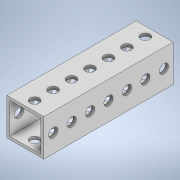
# Autodesk Inventor part: SquareTube
Saved by Autodesk Inventor 2020 (Build 240168000, 168)
## iProperties
Created: 2021-11-12
Part Number: SquareTube
Material: Generic
Document SubType Name: Modeling
Designer: 17185
Density: 1 g/cm^3
Appearance: Default
Author: 17185
Autodesk Inventor part; units mm, degrees
ref_plane "YZ Plane" through (0, 0, 0) normal (1, 0, 0) x (0, 1, 0)
ref_plane "XZ Plane" through (0, 0, 0) normal (0, 1, 0) x (-1, 0, 0)
ref_plane "XY Plane" through (0, 0, 0) normal (0, 0, 1) x (1, 0, 0)
sketch "Sketch1" plane through (0, 0, 0) normal (0, 0, 1) x (1, 0, 0)
  line L0 (-12.7, 12.7) -> (12.7, 12.7)
  line L1 (12.7, 12.7) -> (12.7, -12.7)
  line L2 (12.7, -12.7) -> (-12.7, -12.7)
  line L3 (-12.7, -12.7) -> (-12.7, 12.7)
  line L4 (-12.7, 12.7) -> (12.7, -12.7) construction
  line L5 (12.7, 12.7) -> (-12.7, -12.7) construction
  point P0 (0, 0)
  dimension "d0" = 25.4
  dimension "d1" = 25.4
  constraints: 12 end point, 2 midpoint, 2 parallel, 1 horizontal, 1 perpendicular
  measures "d0" distance of L0.end L1.end
  measures "d1" distance of L1.end L2.end
extrude "Extrusion1" add sketch "Sketch1" along normal blind 88.9
shell "Shell1" thickness 1.9844 removed faces 2 at (4.2333, -4.2333, 0) at (4.2333, -4.2333, 88.9)
sketch "Sketch2" plane through (-12.7, -12.7, 0) normal (-1, 0, 0) x (0, 0, 1)
  circle A0 centre (19.0501, 12.7399) radius 3.175
  circle A1 centre (31.7501, 12.7399) radius 3.175
  line L0 (0, 12.7) -> (88.9, 12.7) construction
  circle A2 centre (44.45, 12.7) radius 3.175
  circle A3 centre (57.15, 12.7) radius 3.175
  circle A4 centre (69.85, 12.7) radius 3.175
  circle A5 centre (82.55, 12.7) radius 3.175
  line L1 (0, 25.4) -> (88.9, 25.4) construction
  line L2 (44.45, 25.4) -> (44.45, 0) construction
  circle A6 centre (6.3501, 12.7) radius 3.175
  dimension "d5" = 6.35
  dimension "d6" = 6.35
  dimension "d7" = 6.35
  dimension "d8" = 6.35
  dimension "d9" = 6.35
  dimension "d10" = 6.35
  dimension "d11" = 12.7
  dimension "d12" = 12.7
  dimension "d13" = 12.7
  dimension "d14" = 12.7
  dimension "d15" = 12.7
  dimension "d16" = 6.35
  dimension "d17" = 12.7
  constraints: 7 centre point, 4 end point, 4 point on line, 3 midpoint, 1 horizontal, 1 vertical
  measures "d5" diameter of A0
  measures "d6" diameter of A1
  measures "d7" diameter of A2
  measures "d8" diameter of A3
  measures "d9" diameter of A4
  measures "d10" diameter of A5
  measures "d11" distance of A1.centre A0.centre
  measures "d12" distance of A2.centre A1.centre
  measures "d13" distance of A2.centre A3.centre
  measures "d14" distance of A4.centre A3.centre
  measures "d15" distance of A5.centre A4.centre
  measures "d16" diameter of A6
  measures "d17" distance of A6.centre A0.centre
extrude "Extrusion2" cut sketch "Sketch2" against normal blind 88.9
sketch "Sketch3" plane through (-12.7, 12.7, 0) normal (0, 1, 0) x (1, 0, 0)
  line L0 (23.4156, -47.625) -> (25.4, -47.625) construction
  circle A0 centre (12.7, -44.45) radius 3.175
  circle A1 centre (12.7, -31.75) radius 3.175
  circle A2 centre (12.7, -19.05) radius 3.175
  circle A3 centre (12.7, -6.35) radius 3.175
  line L1 (12.7, 0) -> (12.7, -88.9) construction
  line L2 (0, -88.9) -> (25.4, -88.9) construction
  line L3 (25.4, -44.45) -> (0, -44.45) construction
  line L4 (0, -47.625) -> (0, -41.275) construction
  circle A4 centre (12.7, -57.15) radius 3.175
  circle A5 centre (12.7, -69.85) radius 3.175
  circle A6 centre (12.7, -82.55) radius 3.175
  line L5 (12.7, -88.9) -> (12.7, 0) construction
  dimension "d20" = 6.35
  dimension "d21" = 6.35
  dimension "d22" = 6.35
  dimension "d23" = 6.35
  dimension "d25" = 12.7
  dimension "d26" = 12.7
  dimension "d27" = 12.7
  constraints: 7 centre point, 6 end point, 5 symmetric about line, 3 midpoint, 1 coincident, 3 other
  measures "d20" diameter of A0
  measures "d21" diameter of A1
  measures "d22" diameter of A2
  measures "d23" diameter of A3
  measures "d25" distance of A1.centre A0.centre
  measures "d26" distance of A2.centre A1.centre
  measures "d27" distance of A3.centre A2.centre
extrude "Extrusion3" cut sketch "Sketch3" against normal blind 88.9
equation "\"d6\" = d5"
equation "\"d7\" = d5"
equation "\"d8\" = d5"
equation "\"d9\" = d5"
equation "\"d10\" = d5"
equation "\"d12\" = d11"
equation "\"d13\" = d11"
equation "\"d14\" = d11"
equation "\"d15\" = d11"
equation "\"d16\" = d5"
equation "\"d17\" = d11"
equation "\"d21\" = d20"
equation "\"d22\" = d20"
equation "\"d23\" = d20"
equation "\"d26\" = d25"
equation "\"d27\" = d25"
body "Solid1"
